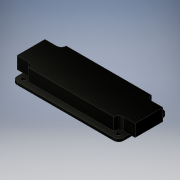
# Autodesk Inventor part: RaspberryPi0W-BerryIMUV3-SafeSpecs
Saved by Autodesk Inventor 2019 (Build 230136000, 136)
## iProperties
Created: 2019-04-03
Part Number: RaspberryPi0W-BerryIMUV3-SafeSpecs
Material: ABS Plastic
Document SubType Name: Modeling
Designer: Epsilon
Density: 1.06 g/cm^3
Appearance: Smooth - White
Author: Epsilon
Autodesk Inventor part; units mm, degrees
ref_plane "YZ Plane" through (0, 0, 0) normal (1, 0, 0) x (0, 1, 0)
ref_plane "XZ Plane" through (0, 0, 0) normal (0, 1, 0) x (-1, 0, 0)
ref_plane "XY Plane" through (0, 0, 0) normal (0, 0, 1) x (1, 0, 0)
sketch "Sketch1" plane through (0, 0, 0) normal (0, 1, 0) x (-1, 0, 0)
  line L0 (3, 0) -> (62, 0)
  line L1 (65, -3) -> (65, -27)
  line L2 (62, -30) -> (3, -30)
  line L3 (0, -27) -> (0, -3)
  arc A0 (65, -3) -> (62, 0) centre (62, -3) ccw
  arc A1 (62, -30) -> (65, -27) centre (62, -27) ccw
  arc A2 (0, -27) -> (3, -30) centre (3, -27) ccw
  arc A3 (3, 0) -> (0, -3) centre (3, -3) ccw
  circle A4 centre (61.5, -26.5) radius 1.25
  circle A5 centre (61.5, -3.5) radius 1.25
  circle A6 centre (3.5, -26.5) radius 1.25
  circle A7 centre (3.5, -3.5) radius 1.25
  point P0 (0, 0)
  point P1 (65, -30)
  point P2 (65, 0)
  point P3 (0, -30)
  dimension "d0" = 65
  dimension "d1" = 30
  dimension "d2" = 3
  dimension "d3" = 2.5
  dimension "d4" = 3.5
  dimension "d5" = 3.5
  dimension "d8" = 23
  dimension "d11" = 58
  constraints: 8 centre point, 8 end point, 8 point on circle, 8 point on line, 8 tangent, 3 equal radius, 2 horizontal, 2 parallel, 1 perpendicular, 1 vertical, 6 other
  measures "d0" distance of point (65, -30) point (0, -30)
  measures "d1" distance of point (65, 0) point (65, -30)
  measures "d2" radius of A0
  measures "d3" diameter of A4
  measures "d4" distance from line of L1 A4.centre
  measures "d5" distance from line of L2 A4.centre
  measures "d8" distance of A4.centre A5.centre
  measures "d11" distance of A4.centre A6.centre
extrude "Extrusion1" add sketch "Sketch1" along normal blind 1.6
sketch "Sketch2" plane through (0, 1.6, 0) normal (0, 1, 0) x (1, 0, 0)
  circle A0 centre (-61.5, 26.5) radius 1.25 projected
  line L0 (-65, 27) -> (-65, 3) construction
  line L1 (-65, 3) -> (-65, 27) construction
  line L2 (-3, 30) -> (-62, 30) construction
  line L3 (-62, 30) -> (-3, 30) construction
  circle A1 centre (-61.5, 26.5) radius 3 construction
  circle A2 centre (-61.5, 3.5) radius 3 construction
  circle A3 centre (-3.5, 26.5) radius 3 construction
  circle A4 centre (-3.5, 3.5) radius 3 construction
  circle A5 centre (-61.5, 3.5) radius 1.25 construction
  line L4 (-3.5, 3.5) -> (-61.5, 3.5) construction
  line L5 (-61.5, 3.5) -> (-61.5, 26.5) construction
  circle A6 centre (-3.5, 26.5) radius 1.25 construction
  line L6 (-61.5, 26.5) -> (-60.25, 26.5) construction
  circle A7 centre (-3.5, 3.5) radius 1.25 construction
  line L7 (-3.5, 26.5) -> (-3.5, 3.5) construction
  line L8 (-61.5, 3.5) -> (-61.5, 26.5) construction
  line L9 (-3.5, 26.5) -> (-61.5, 26.5) construction
  line L10 (-62, 0) -> (-3, 0) construction
  line L11 (-60.25, 26.5) -> (-3.5, 26.5) construction
  line L12 (-61.5, 6.5) -> (-61.5, 23.5)
  line L13 (-58.5, 26.5) -> (-6.5, 26.5)
  line L14 (-3.5, 23.5) -> (-3.5, 6.5)
  line L15 (-6.5, 3.5) -> (-58.5, 3.5)
  arc A8 (-61.5, 23.5) -> (-58.5, 26.5) centre (-61.5, 26.5) ccw
  arc A9 (-6.5, 26.5) -> (-3.5, 23.5) centre (-3.5, 26.5) ccw
  arc A10 (-3.5, 6.5) -> (-6.5, 3.5) centre (-3.5, 3.5) ccw
  arc A11 (-58.5, 3.5) -> (-61.5, 6.5) centre (-61.5, 3.5) ccw
  line L16 (-61.5, 6.5) -> (-68.5, 6.5)
  line L17 (-68.5, 6.5) -> (-68.5, 23.5)
  line L18 (-68.5, 23.5) -> (-61.5, 23.5)
  line L19 (-3.5, 6.5) -> (3.5, 6.5)
  line L20 (3.5, 6.5) -> (3.5, 23.5)
  line L21 (3.5, 23.5) -> (-3.5, 23.5)
  point P0 (0, 0)
  dimension "d17" = 6
  dimension "d20" = 23
  dimension "d23" = 58
  dimension "d28" = 7
  dimension "d29" = 7
  constraints: 38 end point, 16 point on circle, 10 point on line, 9 perpendicular, 8 centre point, 5 collinear, 3 concentric, 2 coincident, 2 horizontal, 2 tangent, 1 horizontal alignment, 1 parallel, 1 vertical, 7 other
  measures "d17" diameter of A1
  measures "d20" distance of L5.end A2.centre
  measures "d23" distance of L5.end A3.centre
  measures "d28" distance of L12.start L16.end
  measures "d29" distance of L14.end L19.end
extrude "Extrusion3" add sketch "Sketch2" along normal blind 7.5 contours L16 L17 L18 L12 | L12 A8 L13 A9 L14 A10 L15 A11 | L14 L21 L20 L19
body "Solid1"
